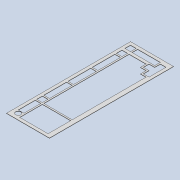
# Autodesk Inventor part: Layout
Saved by Autodesk Inventor 2021 (Build 250183000, 183)
## iProperties
Created: 2021-12-04
Part Number: Layout
Material: Generic
Document SubType Name: Modeling
Designer: Matthew Flooks
Density: 1 g/cm^3
Appearance: Default
Author: Matthew Flooks
Autodesk Inventor part; units mm, degrees
ref_plane "YZ Plane" through (0, 0, 0) normal (1, 0, 0) x (0, 1, 0)
ref_plane "XZ Plane" through (0, 0, 0) normal (0, 1, 0) x (-1, 0, 0)
ref_plane "XY Plane" through (0, 0, 0) normal (0, 0, 1) x (1, 0, 0)
sketch "Sketch1" plane through (0, 0, 0) normal (0, 1, 0) x (-1, 0, 0)
  line L0 (0, 0) -> (18, 0)
  line L1 (18, 0) -> (18, -37.05)
  line L2 (18, -37.05) -> (0, -37.05)
  line L3 (0, -37.05) -> (0, 0)
  line L4 (18, -38.1) -> (0, -38.1)
  line L5 (0, -38.1) -> (0, -56.1)
  line L6 (0, -56.1) -> (18, -56.1)
  line L7 (18, -56.1) -> (18, -38.1)
  line L8 (0, -57.15) -> (37.05, -57.15)
  line L9 (37.05, -57.15) -> (37.05, -75.15)
  line L10 (37.05, -75.15) -> (0, -75.15)
  line L11 (0, -75.15) -> (0, -57.15)
  line L12 (19.05, -56.1) -> (37.05, -56.1)
  line L13 (37.05, -56.1) -> (37.05, -38.1)
  line L14 (37.05, -38.1) -> (19.05, -38.1)
  line L15 (19.05, -38.1) -> (19.05, -56.1)
  line L16 (19.05, -37.05) -> (37.05, -37.05)
  line L17 (37.05, -37.05) -> (37.05, -19.05)
  line L18 (37.05, -19.05) -> (19.05, -19.05)
  line L19 (19.05, -19.05) -> (19.05, -37.05)
  line L20 (19.05, -18) -> (37.05, -18)
  line L21 (37.05, -18) -> (37.05, 0)
  line L22 (37.05, 0) -> (19.05, 0)
  line L23 (19.05, 0) -> (19.05, -18)
  line L24 (38.1, 0) -> (56.1, 0)
  line L25 (56.1, 0) -> (56.1, -18)
  line L26 (56.1, -18) -> (38.1, -18)
  line L27 (38.1, -18) -> (38.1, 0)
  line L28 (38.1, -19.05) -> (56.1, -19.05)
  line L29 (56.1, -19.05) -> (56.1, -37.05)
  line L30 (56.1, -37.05) -> (38.1, -37.05)
  line L31 (38.1, -37.05) -> (38.1, -19.05)
  line L32 (38.1, -38.1) -> (56.1, -38.1)
  line L33 (56.1, -38.1) -> (56.1, -56.1)
  line L34 (56.1, -56.1) -> (38.1, -56.1)
  line L35 (38.1, -56.1) -> (38.1, -38.1)
  line L36 (38.1, -57.15) -> (75.15, -57.15)
  line L37 (75.15, -57.15) -> (75.15, -75.15)
  line L38 (75.15, -75.15) -> (38.1, -75.15)
  line L39 (38.1, -75.15) -> (38.1, -57.15)
  line L40 (57.15, -56.1) -> (75.15, -56.1)
  line L41 (75.15, -56.1) -> (75.15, -38.1)
  line L42 (75.15, -38.1) -> (57.15, -38.1)
  line L43 (57.15, -38.1) -> (57.15, -56.1)
  line L44 (57.15, -37.05) -> (75.15, -37.05)
  line L45 (75.15, -37.05) -> (75.15, -19.05)
  line L46 (75.15, -19.05) -> (57.15, -19.05)
  line L47 (57.15, -19.05) -> (57.15, -37.05)
  line L48 (57.15, -18) -> (75.15, -18)
  line L49 (75.15, -18) -> (75.15, 0)
  line L50 (75.15, 0) -> (57.15, 0)
  line L51 (57.15, 0) -> (57.15, -18)
  line L52 (76.2, 0) -> (94.2, 0)
  line L53 (94.2, 0) -> (94.2, -18)
  line L54 (94.2, -18) -> (76.2, -18)
  line L55 (76.2, -18) -> (76.2, 0)
  line L56 (76.2, -19.05) -> (94.2, -19.05)
  line L57 (94.2, -19.05) -> (94.2, -37.05)
  line L58 (94.2, -37.05) -> (76.2, -37.05)
  line L59 (76.2, -37.05) -> (76.2, -19.05)
  line L60 (76.2, -38.1) -> (94.2, -38.1)
  line L61 (94.2, -38.1) -> (94.2, -56.1)
  line L62 (94.2, -56.1) -> (76.2, -56.1)
  line L63 (76.2, -56.1) -> (76.2, -38.1)
  line L64 (76.2, -57.15) -> (94.2, -57.15)
  line L65 (94.2, -57.15) -> (94.2, -75.15)
  line L66 (94.2, -75.15) -> (76.2, -75.15)
  line L67 (76.2, -75.15) -> (76.2, -57.15)
  line L68 (100.0125, -19.05) -> (118.0125, -19.05)
  line L69 (118.0125, -19.05) -> (118.0125, -37.05)
  line L70 (118.0125, -37.05) -> (100.0125, -37.05)
  line L71 (100.0125, -37.05) -> (100.0125, -19.05)
  line L72 (100.0125, -38.1) -> (118.0125, -38.1)
  line L73 (118.0125, -38.1) -> (118.0125, -56.1)
  line L74 (118.0125, -56.1) -> (100.0125, -56.1)
  line L75 (100.0125, -56.1) -> (100.0125, -38.1)
  line L76 (100.0125, -57.15) -> (118.0125, -57.15)
  line L77 (118.0125, -57.15) -> (118.0125, -75.15)
  line L78 (118.0125, -75.15) -> (100.0125, -75.15)
  line L79 (100.0125, -75.15) -> (100.0125, -57.15)
  line L80 (0, -80.9625) -> (18, -80.9625)
  line L81 (18, -80.9625) -> (18, -103.725)
  line L82 (18, -103.725) -> (0, -103.725)
  line L83 (0, -103.725) -> (0, -80.9625)
  line L84 (0, -104.775) -> (18, -104.775)
  line L85 (18, -104.775) -> (18, -127.5375)
  line L86 (18, -127.5375) -> (0, -127.5375)
  line L87 (0, -127.5375) -> (0, -104.775)
  line L88 (0, -128.5875) -> (18, -128.5875)
  line L89 (18, -128.5875) -> (18, -151.35)
  line L90 (18, -151.35) -> (0, -151.35)
  line L91 (0, -151.35) -> (0, -128.5875)
  line L92 (0, -152.4) -> (18, -152.4)
  line L93 (18, -152.4) -> (18, -270.4)
  line L94 (18, -270.4) -> (0, -270.4)
  line L95 (0, -270.4) -> (0, -152.4)
  line L96 (0, -271.45) -> (18, -271.45)
  line L97 (18, -271.45) -> (18, -289.45)
  line L98 (18, -289.45) -> (0, -289.45)
  line L99 (0, -289.45) -> (0, -271.45)
  line L100 (0, -290.5) -> (18, -290.5)
  line L101 (18, -290.5) -> (18, -308.5)
  line L102 (18, -308.5) -> (0, -308.5)
  line L103 (0, -308.5) -> (0, -290.5)
  line L104 (0, -309.55) -> (18, -309.55)
  line L105 (18, -309.55) -> (18, -327.55)
  line L106 (18, -327.55) -> (0, -327.55)
  line L107 (0, -327.55) -> (0, -309.55)
  line L108 (19.05, -80.9625) -> (37.05, -80.9625)
  line L109 (37.05, -80.9625) -> (37.05, -122.775)
  line L110 (37.05, -122.775) -> (19.05, -122.775)
  line L111 (19.05, -122.775) -> (19.05, -80.9625)
  line L112 (38.1, -80.9625) -> (56.1, -80.9625)
  line L113 (56.1, -80.9625) -> (56.1, -113.25)
  line L114 (56.1, -113.25) -> (38.1, -113.25)
  line L115 (38.1, -113.25) -> (38.1, -80.9625)
  line L116 (57.15, -80.9625) -> (75.15, -80.9625)
  line L117 (75.15, -80.9625) -> (75.15, -108.4875)
  line L118 (75.15, -108.4875) -> (57.15, -108.4875)
  line L119 (57.15, -108.4875) -> (57.15, -80.9625)
  line L120 (76.2, -80.9625) -> (94.2, -80.9625)
  line L121 (94.2, -80.9625) -> (94.2, -98.9625)
  line L122 (94.2, -98.9625) -> (76.2, -98.9625)
  line L123 (76.2, -98.9625) -> (76.2, -80.9625)
  line L124 (19.05, -123.825) -> (37.05, -123.825)
  line L125 (37.05, -123.825) -> (37.05, -141.825)
  line L126 (37.05, -141.825) -> (19.05, -141.825)
  line L127 (19.05, -141.825) -> (19.05, -123.825)
  line L128 (19.05, -142.875) -> (37.05, -142.875)
  line L129 (37.05, -142.875) -> (37.05, -160.875)
  line L130 (37.05, -160.875) -> (19.05, -160.875)
  line L131 (19.05, -160.875) -> (19.05, -142.875)
  line L132 (19.05, -161.925) -> (37.05, -161.925)
  line L133 (37.05, -161.925) -> (37.05, -179.925)
  line L134 (37.05, -179.925) -> (19.05, -179.925)
  line L135 (19.05, -179.925) -> (19.05, -161.925)
  line L136 (19.05, -180.975) -> (37.05, -180.975)
  line L137 (37.05, -180.975) -> (37.05, -198.975)
  line L138 (37.05, -198.975) -> (19.05, -198.975)
  line L139 (19.05, -198.975) -> (19.05, -180.975)
  line L140 (19.05, -200.025) -> (37.05, -200.025)
  line L141 (37.05, -200.025) -> (37.05, -218.025)
  line L142 (37.05, -218.025) -> (19.05, -218.025)
  line L143 (19.05, -218.025) -> (19.05, -200.025)
  line L144 (19.05, -219.075) -> (37.05, -219.075)
  line L145 (37.05, -219.075) -> (37.05, -237.075)
  line L146 (37.05, -237.075) -> (19.05, -237.075)
  line L147 (19.05, -237.075) -> (19.05, -219.075)
  line L148 (19.05, -238.125) -> (37.05, -238.125)
  line L149 (37.05, -238.125) -> (37.05, -256.125)
  line L150 (37.05, -256.125) -> (19.05, -256.125)
  line L151 (19.05, -256.125) -> (19.05, -238.125)
  line L152 (19.05, -257.175) -> (37.05, -257.175)
  line L153 (37.05, -257.175) -> (37.05, -275.175)
  line L154 (37.05, -275.175) -> (19.05, -275.175)
  line L155 (19.05, -275.175) -> (19.05, -257.175)
  line L156 (19.05, -276.225) -> (37.05, -276.225)
  line L157 (37.05, -276.225) -> (37.05, -294.225)
  line L158 (37.05, -294.225) -> (19.05, -294.225)
  line L159 (19.05, -294.225) -> (19.05, -276.225)
  line L160 (19.05, -313.275) -> (37.05, -313.275)
  line L161 (37.05, -313.275) -> (37.05, -295.275)
  line L162 (37.05, -295.275) -> (19.05, -295.275)
  line L163 (19.05, -295.275) -> (19.05, -313.275)
  line L164 (19.05, -314.325) -> (37.05, -314.325)
  line L165 (37.05, -314.325) -> (37.05, -346.6125)
  line L166 (37.05, -346.6125) -> (19.05, -346.6125)
  line L167 (19.05, -346.6125) -> (19.05, -314.325)
  line L168 (38.1, -114.3) -> (56.1, -114.3)
  line L169 (56.1, -114.3) -> (56.1, -132.3)
  line L170 (56.1, -132.3) -> (38.1, -132.3)
  line L171 (38.1, -132.3) -> (38.1, -114.3)
  line L172 (38.1, -133.35) -> (56.1, -133.35)
  line L173 (56.1, -133.35) -> (56.1, -151.35)
  line L174 (56.1, -151.35) -> (38.1, -151.35)
  line L175 (38.1, -151.35) -> (38.1, -133.35)
  line L176 (38.1, -152.4) -> (56.1, -152.4)
  line L177 (56.1, -152.4) -> (56.1, -170.4)
  line L178 (56.1, -170.4) -> (38.1, -170.4)
  line L179 (38.1, -170.4) -> (38.1, -152.4)
  line L180 (38.1, -171.45) -> (56.1, -171.45)
  line L181 (56.1, -171.45) -> (56.1, -189.45)
  line L182 (56.1, -189.45) -> (38.1, -189.45)
  line L183 (38.1, -189.45) -> (38.1, -171.45)
  line L184 (38.1, -190.5) -> (56.1, -190.5)
  line L185 (56.1, -190.5) -> (56.1, -208.5)
  line L186 (56.1, -208.5) -> (38.1, -208.5)
  line L187 (38.1, -208.5) -> (38.1, -190.5)
  line L188 (56.1, -209.55) -> (38.1, -209.55)
  line L189 (38.1, -209.55) -> (38.1, -227.55)
  line L190 (38.1, -227.55) -> (56.1, -227.55)
  line L191 (56.1, -227.55) -> (56.1, -209.55)
  line L192 (38.1, -228.6) -> (56.1, -228.6)
  line L193 (56.1, -228.6) -> (56.1, -246.6)
  line L194 (56.1, -246.6) -> (38.1, -246.6)
  line L195 (38.1, -246.6) -> (38.1, -228.6)
  line L196 (38.1, -247.65) -> (56.1, -247.65)
  line L197 (56.1, -247.65) -> (56.1, -265.65)
  line L198 (56.1, -265.65) -> (38.1, -265.65)
  line L199 (38.1, -265.65) -> (38.1, -247.65)
  line L200 (38.1, -266.7) -> (56.1, -266.7)
  line L201 (56.1, -266.7) -> (56.1, -284.7)
  line L202 (56.1, -284.7) -> (38.1, -284.7)
  line L203 (38.1, -284.7) -> (38.1, -266.7)
  line L204 (38.1, -285.75) -> (56.1, -285.75)
  line L205 (56.1, -285.75) -> (56.1, -303.75)
  line L206 (56.1, -303.75) -> (38.1, -303.75)
  line L207 (38.1, -303.75) -> (38.1, -285.75)
  line L208 (38.1, -304.8) -> (56.1, -304.8)
  line L209 (56.1, -304.8) -> (56.1, -322.8)
  line L210 (56.1, -322.8) -> (38.1, -322.8)
  line L211 (38.1, -322.8) -> (38.1, -304.8)
  line L212 (38.1, -323.85) -> (56.1, -323.85)
  line L213 (56.1, -323.85) -> (56.1, -365.6625)
  line L214 (56.1, -365.6625) -> (38.1, -365.6625)
  line L215 (38.1, -365.6625) -> (38.1, -323.85)
  line L216 (75.15, -109.5375) -> (57.15, -109.5375)
  line L217 (57.15, -109.5375) -> (57.15, -127.5375)
  line L218 (57.15, -127.5375) -> (75.15, -127.5375)
  line L219 (75.15, -127.5375) -> (75.15, -109.5375)
  line L220 (75.15, -128.5875) -> (57.15, -128.5875)
  line L221 (57.15, -128.5875) -> (57.15, -146.5875)
  line L222 (57.15, -146.5875) -> (75.15, -146.5875)
  line L223 (75.15, -146.5875) -> (75.15, -128.5875)
  line L224 (75.15, -147.6375) -> (57.15, -147.6375)
  line L225 (57.15, -147.6375) -> (57.15, -165.6375)
  line L226 (57.15, -165.6375) -> (75.15, -165.6375)
  line L227 (75.15, -165.6375) -> (75.15, -147.6375)
  line L228 (75.15, -166.6875) -> (57.15, -166.6875)
  line L229 (57.15, -166.6875) -> (57.15, -184.6875)
  line L230 (57.15, -184.6875) -> (75.15, -184.6875)
  line L231 (75.15, -184.6875) -> (75.15, -166.6875)
  line L232 (75.15, -185.7375) -> (57.15, -185.7375)
  line L233 (57.15, -185.7375) -> (57.15, -203.7375)
  line L234 (57.15, -203.7375) -> (75.15, -203.7375)
  line L235 (75.15, -203.7375) -> (75.15, -185.7375)
  line L236 (75.15, -204.7875) -> (57.15, -204.7875)
  line L237 (57.15, -204.7875) -> (57.15, -222.7875)
  line L238 (57.15, -222.7875) -> (75.15, -222.7875)
  line L239 (75.15, -222.7875) -> (75.15, -204.7875)
  line L240 (75.15, -223.8375) -> (57.15, -223.8375)
  line L241 (57.15, -223.8375) -> (57.15, -241.8375)
  line L242 (57.15, -241.8375) -> (75.15, -241.8375)
  line L243 (75.15, -241.8375) -> (75.15, -223.8375)
  line L244 (75.15, -242.8875) -> (57.15, -242.8875)
  line L245 (57.15, -242.8875) -> (57.15, -260.8875)
  line L246 (57.15, -260.8875) -> (75.15, -260.8875)
  line L247 (75.15, -260.8875) -> (75.15, -242.8875)
  line L248 (75.15, -261.9375) -> (57.15, -261.9375)
  line L249 (57.15, -261.9375) -> (57.15, -279.9375)
  line L250 (57.15, -279.9375) -> (75.15, -279.9375)
  line L251 (75.15, -279.9375) -> (75.15, -261.9375)
  line L252 (75.15, -280.9875) -> (57.15, -280.9875)
  line L253 (57.15, -280.9875) -> (57.15, -298.9875)
  line L254 (57.15, -298.9875) -> (75.15, -298.9875)
  line L255 (75.15, -298.9875) -> (75.15, -280.9875)
  line L256 (57.15, -300.0375) -> (75.15, -300.0375)
  line L257 (75.15, -300.0375) -> (75.15, -318.0375)
  line L258 (75.15, -318.0375) -> (57.15, -318.0375)
  line L259 (57.15, -318.0375) -> (57.15, -300.0375)
  line L260 (57.15, -319.0875) -> (75.15, -319.0875)
  line L261 (75.15, -319.0875) -> (75.15, -337.0875)
  line L262 (75.15, -337.0875) -> (57.15, -337.0875)
  line L263 (57.15, -337.0875) -> (57.15, -319.0875)
  line L264 (75.15, -338.1375) -> (57.15, -338.1375)
  line L265 (57.15, -338.1375) -> (57.15, -365.6625)
  line L266 (57.15, -365.6625) -> (75.15, -365.6625)
  line L267 (75.15, -365.6625) -> (75.15, -338.1375)
  line L268 (76.2, -100.0125) -> (94.2, -100.0125)
  line L269 (94.2, -100.0125) -> (94.2, -118.0125)
  line L270 (94.2, -118.0125) -> (76.2, -118.0125)
  line L271 (76.2, -118.0125) -> (76.2, -100.0125)
  line L272 (76.2, -119.0625) -> (94.2, -119.0625)
  line L273 (94.2, -119.0625) -> (94.2, -137.0625)
  line L274 (94.2, -137.0625) -> (76.2, -137.0625)
  line L275 (76.2, -137.0625) -> (76.2, -119.0625)
  line L276 (76.2, -138.1125) -> (94.2, -138.1125)
  line L277 (94.2, -138.1125) -> (94.2, -156.1125)
  line L278 (94.2, -156.1125) -> (76.2, -156.1125)
  line L279 (76.2, -156.1125) -> (76.2, -138.1125)
  line L280 (76.2, -157.1625) -> (94.2, -157.1625)
  line L281 (94.2, -157.1625) -> (94.2, -175.1625)
  line L282 (94.2, -175.1625) -> (76.2, -175.1625)
  line L283 (76.2, -175.1625) -> (76.2, -157.1625)
  line L284 (76.2, -176.2125) -> (94.2, -176.2125)
  line L285 (94.2, -176.2125) -> (94.2, -194.2125)
  line L286 (94.2, -194.2125) -> (76.2, -194.2125)
  line L287 (76.2, -194.2125) -> (76.2, -176.2125)
  line L288 (76.2, -195.2625) -> (94.2, -195.2625)
  line L289 (94.2, -195.2625) -> (94.2, -213.2625)
  line L290 (94.2, -213.2625) -> (76.2, -213.2625)
  line L291 (76.2, -213.2625) -> (76.2, -195.2625)
  line L292 (76.2, -214.3125) -> (94.2, -214.3125)
  line L293 (94.2, -214.3125) -> (94.2, -232.3125)
  line L294 (94.2, -232.3125) -> (76.2, -232.3125)
  line L295 (76.2, -232.3125) -> (76.2, -214.3125)
  line L296 (76.2, -233.3625) -> (94.2, -233.3625)
  line L297 (94.2, -233.3625) -> (94.2, -251.3625)
  line L298 (94.2, -251.3625) -> (76.2, -251.3625)
  line L299 (76.2, -251.3625) -> (76.2, -233.3625)
  line L300 (76.2, -252.4125) -> (94.2, -252.4125)
  line L301 (94.2, -252.4125) -> (94.2, -270.4125)
  line L302 (94.2, -270.4125) -> (76.2, -270.4125)
  line L303 (76.2, -270.4125) -> (76.2, -252.4125)
  line L304 (76.2, -271.4625) -> (94.2, -271.4625)
  line L305 (94.2, -271.4625) -> (94.2, -289.4625)
  line L306 (94.2, -289.4625) -> (76.2, -289.4625)
  line L307 (76.2, -289.4625) -> (76.2, -271.4625)
  line L308 (76.2, -290.5125) -> (94.2, -290.5125)
  line L309 (94.2, -290.5125) -> (94.2, -308.5125)
  line L310 (94.2, -308.5125) -> (76.2, -308.5125)
  line L311 (76.2, -308.5125) -> (76.2, -290.5125)
  line L312 (76.2, -309.5625) -> (94.2, -309.5625)
  line L313 (94.2, -309.5625) -> (94.2, -327.5625)
  line L314 (94.2, -327.5625) -> (76.2, -327.5625)
  line L315 (76.2, -327.5625) -> (76.2, -309.5625)
  line L316 (76.2, -328.6125) -> (94.2, -328.6125)
  line L317 (94.2, -328.6125) -> (94.2, -365.6625)
  line L318 (94.2, -365.6625) -> (76.2, -365.6625)
  line L319 (76.2, -365.6625) -> (76.2, -328.6125)
  line L320 (100.0125, -80.9625) -> (118.0125, -80.9625)
  line L321 (118.0125, -80.9625) -> (118.0125, -98.9625)
  line L322 (118.0125, -98.9625) -> (100.0125, -98.9625)
  line L323 (100.0125, -98.9625) -> (100.0125, -80.9625)
  line L324 (118.0125, -104.775) -> (100.0125, -104.775)
  line L325 (100.0125, -104.775) -> (100.0125, -122.775)
  line L326 (100.0125, -122.775) -> (118.0125, -122.775)
  line L327 (118.0125, -122.775) -> (118.0125, -104.775)
  line L328 (118.0125, -123.825) -> (100.0125, -123.825)
  line L329 (100.0125, -123.825) -> (100.0125, -141.825)
  line L330 (100.0125, -141.825) -> (118.0125, -141.825)
  line L331 (118.0125, -141.825) -> (118.0125, -123.825)
  line L332 (118.0125, -142.875) -> (100.0125, -142.875)
  line L333 (100.0125, -142.875) -> (100.0125, -160.875)
  line L334 (100.0125, -160.875) -> (118.0125, -160.875)
  line L335 (118.0125, -160.875) -> (118.0125, -142.875)
  line L336 (118.0125, -161.925) -> (100.0125, -161.925)
  line L337 (100.0125, -161.925) -> (100.0125, -179.925)
  line L338 (100.0125, -179.925) -> (118.0125, -179.925)
  line L339 (118.0125, -179.925) -> (118.0125, -161.925)
  line L340 (118.0125, -203.7375) -> (100.0125, -203.7375)
  line L341 (100.0125, -203.7375) -> (100.0125, -185.7375)
  line L342 (100.0125, -185.7375) -> (118.0125, -185.7375)
  line L343 (118.0125, -185.7375) -> (118.0125, -203.7375)
  line L344 (118.0125, -204.7875) -> (100.0125, -204.7875)
  line L345 (100.0125, -204.7875) -> (100.0125, -222.7875)
  line L346 (100.0125, -222.7875) -> (118.0125, -222.7875)
  line L347 (118.0125, -222.7875) -> (118.0125, -204.7875)
  line L348 (118.0125, -223.8375) -> (100.0125, -223.8375)
  line L349 (100.0125, -223.8375) -> (100.0125, -241.8375)
  line L350 (100.0125, -241.8375) -> (118.0125, -241.8375)
  line L351 (118.0125, -241.8375) -> (118.0125, -223.8375)
  line L352 (118.0125, -242.8875) -> (100.0125, -242.8875)
  line L353 (100.0125, -242.8875) -> (100.0125, -260.8875)
  line L354 (100.0125, -260.8875) -> (118.0125, -260.8875)
  line L355 (118.0125, -260.8875) -> (118.0125, -242.8875)
  line L356 (118.0125, -266.7) -> (100.0125, -266.7)
  line L357 (100.0125, -266.7) -> (100.0125, -284.7)
  line L358 (100.0125, -284.7) -> (118.0125, -284.7)
  line L359 (118.0125, -284.7) -> (118.0125, -266.7)
  line L360 (118.0125, -285.75) -> (100.0125, -285.75)
  line L361 (100.0125, -285.75) -> (100.0125, -303.75)
  line L362 (100.0125, -303.75) -> (118.0125, -303.75)
  line L363 (118.0125, -303.75) -> (118.0125, -285.75)
  line L364 (118.0125, -304.8) -> (100.0125, -304.8)
  line L365 (100.0125, -304.8) -> (100.0125, -322.8)
  line L366 (100.0125, -322.8) -> (118.0125, -322.8)
  line L367 (118.0125, -322.8) -> (118.0125, -304.8)
  line L368 (118.0125, -323.85) -> (100.0125, -323.85)
  line L369 (100.0125, -323.85) -> (100.0125, -341.85)
  line L370 (100.0125, -341.85) -> (118.0125, -341.85)
  line L371 (118.0125, -341.85) -> (118.0125, -323.85)
  line L372 (118.0125, -347.6625) -> (100.0125, -347.6625)
  line L373 (100.0125, -347.6625) -> (100.0125, -365.6625)
  line L374 (100.0125, -365.6625) -> (118.0125, -365.6625)
  line L375 (118.0125, -365.6625) -> (118.0125, -347.6625)
  line L376 (118.0125, -376.2375) -> (100.0125, -376.2375)
  line L377 (100.0125, -376.2375) -> (100.0125, -394.2375)
  line L378 (100.0125, -394.2375) -> (118.0125, -394.2375)
  line L379 (118.0125, -394.2375) -> (118.0125, -376.2375)
  line L380 (13.2375, -333.375) -> (-4.7625, -333.375)
  line L381 (-4.7625, -333.375) -> (-4.7625, -351.375)
  line L382 (-4.7625, -351.375) -> (13.2375, -351.375)
  line L383 (13.2375, -351.375) -> (13.2375, -333.375)
  line L384 (13.2375, -352.425) -> (-4.7625, -352.425)
  line L385 (-4.7625, -352.425) -> (-4.7625, -370.425)
  line L386 (-4.7625, -370.425) -> (13.2375, -370.425)
  line L387 (13.2375, -370.425) -> (13.2375, -352.425)
  line L388 (13.2375, -371.475) -> (-4.7625, -371.475)
  line L389 (-4.7625, -371.475) -> (-4.7625, -389.475)
  line L390 (-4.7625, -389.475) -> (13.2375, -389.475)
  line L391 (13.2375, -389.475) -> (13.2375, -371.475)
  line L392 (14.2875, -370.425) -> (32.2875, -370.425)
  line L393 (32.2875, -370.425) -> (32.2875, -352.425)
  line L394 (32.2875, -352.425) -> (14.2875, -352.425)
  line L395 (14.2875, -352.425) -> (14.2875, -370.425)
  line L396 (19.05, -376.2375) -> (37.05, -376.2375)
  line L397 (37.05, -376.2375) -> (37.05, -394.2375)
  line L398 (37.05, -394.2375) -> (19.05, -394.2375)
  line L399 (19.05, -394.2375) -> (19.05, -376.2375)
  line L400 (57.15, -376.2375) -> (75.15, -376.2375)
  line L401 (75.15, -376.2375) -> (75.15, -394.2375)
  line L402 (75.15, -394.2375) -> (57.15, -394.2375)
  line L403 (57.15, -394.2375) -> (57.15, -376.2375)
  line L404 (76.2, -376.2375) -> (94.2, -376.2375)
  line L405 (94.2, -376.2375) -> (94.2, -394.2375)
  line L406 (94.2, -394.2375) -> (76.2, -394.2375)
  line L407 (76.2, -394.2375) -> (76.2, -376.2375)
  line L408 (56.1, -376.2375) -> (38.1, -376.2375)
  line L409 (38.1, -376.2375) -> (38.1, -394.2375)
  line L410 (38.1, -394.2375) -> (56.1, -394.2375)
  line L411 (56.1, -394.2375) -> (56.1, -376.2375)
  circle A0 centre (109.0125, -9) radius 8.5
  circle A1 centre (109.0125, -9) radius 8.75
  line L412 (118.5125, -18.55) -> (99.5125, -18.55)
  line L413 (99.5125, -18.55) -> (99.5125, -75.65)
  line L414 (99.5125, -75.65) -> (118.5125, -75.65)
  line L415 (118.5125, -75.65) -> (118.5125, -18.55)
  line L416 (118.5125, -80.4625) -> (99.5125, -80.4625)
  line L417 (99.5125, -80.4625) -> (99.5125, -99.4625)
  line L418 (99.5125, -99.4625) -> (118.5125, -99.4625)
  line L419 (118.5125, -99.4625) -> (118.5125, -80.4625)
  line L420 (118.5125, -104.275) -> (99.5125, -104.275)
  line L421 (99.5125, -104.275) -> (99.5125, -180.425)
  line L422 (99.5125, -180.425) -> (118.5125, -180.425)
  line L423 (118.5125, -180.425) -> (118.5125, -104.275)
  line L424 (118.5125, -185.2375) -> (99.5125, -185.2375)
  line L425 (99.5125, -185.2375) -> (99.5125, -261.3875)
  line L426 (99.5125, -261.3875) -> (118.5125, -261.3875)
  line L427 (118.5125, -261.3875) -> (118.5125, -185.2375)
  line L428 (118.5125, -266.2) -> (99.5125, -266.2)
  line L429 (99.5125, -266.2) -> (99.5125, -342.35)
  line L430 (99.5125, -342.35) -> (118.5125, -342.35)
  line L431 (118.5125, -342.35) -> (118.5125, -266.2)
  line L432 (118.5125, -347.1625) -> (99.5125, -347.1625)
  line L433 (99.5125, -347.1625) -> (99.5125, -366.1625)
  line L434 (99.5125, -366.1625) -> (118.5125, -366.1625)
  line L435 (118.5125, -366.1625) -> (118.5125, -347.1625)
  line L436 (118.5125, -375.7375) -> (99.5125, -375.7375)
  line L437 (99.5125, -375.7375) -> (99.5125, -394.7375)
  line L438 (99.5125, -394.7375) -> (118.5125, -394.7375)
  line L439 (118.5125, -394.7375) -> (118.5125, -375.7375)
  line L440 (94.7, -375.7375) -> (18.55, -375.7375)
  line L441 (18.55, -375.7375) -> (18.55, -394.7375)
  line L442 (18.55, -394.7375) -> (94.7, -394.7375)
  line L443 (94.7, -394.7375) -> (94.7, -375.7375)
  line L444 (94.7, 0.5) -> (-0.5, 0.5)
  line L445 (-0.5, 0.5) -> (-0.5, -75.65)
  line L446 (-0.5, -75.65) -> (94.7, -75.65)
  line L447 (94.7, -75.65) -> (94.7, 0.5)
  line L448 (94.7, -80.4625) -> (-0.5, -80.4625)
  line L449 (-0.5, -80.4625) -> (-0.5, -328.05)
  line L450 (-0.5, -328.05) -> (18.55, -328.05)
  line L451 (18.55, -328.05) -> (18.55, -347.1125)
  line L452 (18.55, -347.1125) -> (37.6, -347.1125)
  line L453 (37.6, -347.1125) -> (37.6, -366.1625)
  line L454 (37.6, -366.1625) -> (94.7, -366.1625)
  line L455 (94.7, -366.1625) -> (94.7, -80.4625)
  line L456 (-5.2625, -332.875) -> (-5.2625, -389.975)
  line L457 (-5.2625, -389.975) -> (13.7375, -389.975)
  line L458 (13.7375, -389.975) -> (13.7375, -370.925)
  line L459 (13.7375, -370.925) -> (32.7875, -370.925)
  line L460 (32.7875, -370.925) -> (32.7875, -351.925)
  line L461 (32.7875, -351.925) -> (13.7375, -351.925)
  line L462 (13.7375, -351.925) -> (13.7375, -332.875)
  line L463 (13.7375, -332.875) -> (-5.2625, -332.875)
  line L464 (-15.2625, 10.5) -> (128.5125, 10.5)
  line L465 (128.5125, 10.5) -> (128.5125, -404.7375)
  line L466 (128.5125, -404.7375) -> (-15.2625, -404.7375)
  line L467 (-15.2625, -404.7375) -> (-15.2625, 10.5)
  point P0 (0, 0)
  dimension "d0" = 37.05
  dimension "d1" = 18
  dimension "d2" = 0
  dimension "d3" = 0
  dimension "d4" = 18
  dimension "d5" = 1.05
  dimension "d6" = 37.05
  dimension "d7" = 18
  dimension "d8" = 1.05
  dimension "d10" = 18
  dimension "d12" = 18
  dimension "d13" = 18
  dimension "d15" = 18
  dimension "d16" = 18
  dimension "d17" = 1.05
  dimension "d18" = 1.05
  dimension "d21" = 18
  dimension "d25" = 1.05
  dimension "d26" = 37.05
  dimension "d27" = 18
  dimension "d33" = 1.05
  dimension "d34" = 18
  dimension "d37" = 22.7625
  dimension "d38" = 5.8125
  dimension "d39" = 22.7625
  dimension "d40" = 22.7625
  dimension "d41" = 1.05
  dimension "d42" = 1.05
  dimension "d43" = 1.05
  dimension "d44" = 1.05
  dimension "d45" = 1.05
  dimension "d46" = 1.05
  dimension "d47" = 18
  dimension "d48" = 18
  dimension "d49" = 18
  dimension "d50" = 118
  dimension "d51" = 41.8125
  dimension "d52" = 1.05
  dimension "d53" = 32.2875
  dimension "d54" = 27.525
  dimension "d55" = 18
  dimension "d56" = 1.05
  dimension "d57" = 1.05
  dimension "d58" = 1.05
  dimension "d59" = 1.05
  dimension "d60" = 1.05
  dimension "d61" = 1.05
  dimension "d62" = 1.05
  dimension "d63" = 1.05
  dimension "d64" = 1.05
  dimension "d66" = 18
  dimension "d67" = 18
  dimension "d68" = 18
  dimension "d69" = 18
  dimension "d70" = 18
  dimension "d71" = 18
  dimension "d72" = 18
  dimension "d73" = 18
  dimension "d74" = 18
  dimension "d75" = 18
  dimension "d76" = 1.05
  dimension "d77" = 1.05
  dimension "d78" = 32.2875
  dimension "d79" = 18
  constraints: 936 end point, 228 parallel, 153 point on line, 124 perpendicular, 115 horizontal, 76 collinear, 2 centre point, 1 coincident
  measures "d0" distance of L2.end L0.start
  measures "d1" distance of L1.end L2.end
  measures "d2" distance from line of point (0, 0) L0
  measures "d3" distance from line of point (0, 0) L3
  measures "d4" distance of L4.end L5.end
  measures "d5" distance between parallel lines of L2 L4
  measures "d6" distance of L9.end L10.end
  measures "d7" distance of L10.end L8.start
  measures "d8" distance between parallel lines of L6 L8
  measures "d10" distance of L12.end L13.end
  measures "d12" distance of L17.end L18.end
  measures "d13" distance of L16.end L17.end
  measures "d15" distance of L20.end L21.end
  measures "d16" distance of L21.end L22.end
  measures "d17" distance between parallel lines of L1 L23
  measures "d18" distance between parallel lines of L18 L20
  measures "d21" distance of L24.start L24.end
  measures "d25" distance between parallel lines of L21 L27
  measures "d26" distance of L37.end L38.end
  measures "d27" distance of L41.end L42.end
  measures "d33" distance between parallel lines of L41 L63
  measures "d34" distance of L52.start L52.end
  measures "d37" distance of L82.end L80.start
  measures "d38" distance between parallel lines of L10 L80
  measures "d39" distance of L86.end L84.start
  measures "d40" distance of L90.end L88.start
  measures "d41" distance between parallel lines of L82 L84
  measures "d42" distance between parallel lines of L88 L86
  measures "d43" distance between parallel lines of L92 L90
  measures "d44" distance between parallel lines of L96 L94
  measures "d45" distance between parallel lines of L100 L98
  measures "d46" distance between parallel lines of L104 L102
  measures "d47" distance of L98.end L96.start
  measures "d48" distance of L102.end L100.start
  measures "d49" distance of L106.end L104.start
  measures "d50" distance of L94.end L92.start
  measures "d51" distance of L110.end L108.start
  measures "d52" distance between parallel lines of L111 L81
  measures "d53" distance of L114.end L112.start
  measures "d54" distance of L118.end L116.start
  measures "d55" distance of L122.end L120.start
  measures "d56" distance between parallel lines of L124 L110
  measures "d57" distance between parallel lines of L128 L126
  measures "d58" distance between parallel lines of L132 L130
  measures "d59" distance between parallel lines of L136 L134
  measures "d60" distance between parallel lines of L140 L138
  measures "d61" distance between parallel lines of L144 L142
  measures "d62" distance between parallel lines of L148 L146
  measures "d63" distance between parallel lines of L152 L150
  measures "d64" distance between parallel lines of L156 L154
  measures "d66" distance of L126.end L124.start
  measures "d67" distance of L130.end L128.start
  measures "d68" distance of L134.end L132.start
  measures "d69" distance of L138.end L136.start
  measures "d70" distance of L142.end L140.start
  measures "d71" distance of L146.end L144.start
  measures "d72" distance of L150.end L148.start
  measures "d73" distance of L154.end L152.start
  measures "d74" distance of L158.end L156.start
  measures "d75" distance of L162.end L160.start
  measures "d76" distance between parallel lines of L158 L162
  measures "d77" distance between parallel lines of L160 L164
  measures "d78" distance of L166.end L164.start
  measures "d79" distance of L168.end L169.end
extrude "Extrusion1" add sketch "Sketch1" along normal blind 1 contours L464 L465 L466 L467
equation "\"d0\" = u2"
equation "\"d1\" = u1"
equation "\"d4\" = u1"
equation "\"d5\" = spacing"
equation "\"d6\" = u2"
equation "\"d7\" = u1"
equation "\"d8\" = spacing"
equation "\"d10\" = u1"
equation "\"d12\" = u1"
equation "\"d13\" = u1"
equation "\"d15\" = u1"
equation "\"d16\" = u1"
equation "\"d17\" = spacing"
equation "\"d18\" = spacing"
equation "\"d21\" = u1"
equation "\"d25\" = spacing"
equation "\"d26\" = u2"
equation "\"d27\" = u1"
equation "\"d33\" = spacing"
equation "\"d34\" = u1"
equation "\"d37\" = u125"
equation "\"d39\" = u125"
equation "\"d40\" = u125"
equation "\"d41\" = spacing"
equation "\"d42\" = spacing"
equation "\"d43\" = spacing"
equation "\"d44\" = spacing"
equation "\"d45\" = spacing"
equation "\"d46\" = spacing"
equation "\"d47\" = u1"
equation "\"d48\" = u1"
equation "\"d49\" = u1"
equation "\"d50\" = uspace"
equation "\"d51\" = u225"
equation "\"d52\" = spacing"
equation "\"d53\" = u175"
equation "\"d54\" = u15"
equation "\"d55\" = u1"
equation "\"d56\" = spacing"
equation "\"d57\" = spacing"
equation "\"d58\" = spacing"
equation "\"d59\" = spacing"
equation "\"d60\" = spacing"
equation "\"d61\" = spacing"
equation "\"d62\" = spacing"
equation "\"d63\" = spacing"
equation "\"d64\" = spacing"
equation "\"d66\" = u1"
equation "\"d67\" = u1"
equation "\"d68\" = u1"
equation "\"d69\" = u1"
equation "\"d70\" = u1"
equation "\"d71\" = u1"
equation "\"d72\" = u1"
equation "\"d73\" = u1"
equation "\"d74\" = u1"
equation "\"d75\" = u1"
equation "\"d76\" = spacing"
equation "\"d77\" = spacing"
equation "\"d78\" = u175"
equation "\"d79\" = u1"
equation "\"u2\" = 37.05"
equation "\"u1\" = 18"
equation "\"u125\" = 22.7625"
equation "\"u15\" = 27.525"
equation "\"u175\" = 32.2875"
equation "\"u225\" = 41.8125"
equation "\"u25\" = 46.575"
equation "\"u275\" = 51.3375"
equation "\"spacing\" = 1.05"
equation "\"uspace\" = 118"
equation "\"spacing2\" = 5.8125"
equation "\"size\" = 19.05"
equation "\"gap\" = 0.5"
body "Solid1"
